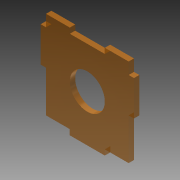
# Autodesk Inventor part: SideB
Saved by Autodesk Inventor 2014 (Build 180170000, 170)
## iProperties
Created: 2014-11-21
Part Number: SideB
Material: Generic
Document SubType Name: Modeling
Designer: JLM
Density: 1 g/cm^3
Appearance: Default
Author: JLM
Autodesk Inventor part; units mm, degrees
ref_plane "YZ Plane" through (0, 0, 0) normal (1, 0, 0) x (0, 1, 0)
ref_plane "XZ Plane" through (0, 0, 0) normal (0, 1, 0) x (-1, 0, 0)
ref_plane "XY Plane" through (0, 0, 0) normal (0, 0, 1) x (1, 0, 0)
sketch "Sketch1" plane through (0, 0, 0) normal (0, 0, 1) x (1, 0, 0)
  line L0 (-25.4, -25.4) -> (25.4, -25.4)
  line L1 (25.4, -25.4) -> (25.4, 25.4)
  line L2 (25.4, 25.4) -> (-25.4, 25.4)
  line L3 (-25.4, 25.4) -> (-25.4, -25.4)
  line L4 (-25.4, -25.4) -> (25.4, 25.4) construction
  line L5 (25.4, -25.4) -> (-25.4, 25.4) construction
  point P0 (0, 0)
  dimension "d0" = 50.8
  dimension "d1" = 50.8
  constraints: 12 end point, 2 midpoint, 2 parallel, 1 horizontal, 1 perpendicular
  measures "d0" distance of L2.end L1.end
  measures "d1" distance of L1.end L0.end
extrude "Extrusion1" add sketch "Sketch1" against normal blind 2.921
sketch "Sketch4" plane through (0, 0, 0) normal (0, 0, 1) x (1, 0, 0)
  line L0 (-25.4, -25.4) -> (-9.525, -25.4)
  line L1 (-9.525, -25.4) -> (-9.525, -22.479)
  line L2 (-9.525, -22.479) -> (-25.4, -22.479)
  line L3 (-25.4, -22.479) -> (-25.4, -25.4)
  line L4 (25.4, 25.4) -> (-25.4, 25.4) projected
  line L5 (-25.4, 25.4) -> (-25.4, -25.4) projected
  line L6 (-9.525, 25.4) -> (9.525, 25.4)
  line L7 (9.525, 25.4) -> (9.525, 22.479)
  line L8 (9.525, 22.479) -> (-9.525, 22.479)
  line L9 (-9.525, 22.479) -> (-9.525, 25.4)
  line L10 (-25.4, -25.4) -> (-22.479, -25.4)
  line L11 (-22.479, -25.4) -> (-22.479, 0)
  line L12 (-22.479, 0) -> (-25.4, 0)
  line L13 (-25.4, 0) -> (-25.4, -25.4)
  line L14 (-25.4, 25.4) -> (-22.479, 25.4)
  line L15 (-22.479, 25.4) -> (-22.479, 19.05)
  line L16 (-22.479, 19.05) -> (-25.4, 19.05)
  line L17 (-25.4, 19.05) -> (-25.4, 25.4)
  line L18 (0, -3.175) -> (0, -6.3407)
  line L19 (25.4, -25.4) -> (9.525, -25.4)
  line L20 (9.525, -25.4) -> (9.525, -22.479)
  line L21 (9.525, -22.479) -> (25.4, -22.479)
  line L22 (25.4, -22.479) -> (25.4, -25.4)
  line L23 (25.4, 25.4) -> (25.4, -25.4)
  line L24 (9.525, 22.479) -> (9.525, 25.4)
  line L25 (25.4, -25.4) -> (22.479, -25.4)
  line L26 (22.479, -25.4) -> (22.479, 0)
  line L27 (22.479, 0) -> (25.4, 0)
  line L28 (25.4, 0) -> (25.4, -25.4)
  line L29 (25.4, 25.4) -> (22.479, 25.4)
  line L30 (22.479, 25.4) -> (22.479, 19.05)
  line L31 (22.479, 19.05) -> (25.4, 19.05)
  line L32 (25.4, 19.05) -> (25.4, 25.4)
  point P0 (0, 0)
  point P1 (25.4, 0.1976)
  dimension "d16" = 2.921
  dimension "d37" = 9.525
  dimension "d38" = 15.875
  dimension "d44" = 2.921
  dimension "d45" = 19.05
  dimension "d46" = 15.875
  dimension "d53" = 25.4
  dimension "d54" = 19.05
  dimension "d55" = 2.921
  dimension "d56" = 2.921
  constraints: 62 end point, 11 symmetric about line, 9 parallel, 4 horizontal, 4 perpendicular, 2 point on line
  measures "d16" distance of L0.end L1.end
  measures "d37" distance from line of point (0, 0) L1
  measures "d38" distance of L0.start L0.end
  measures "d44" distance of L8.end L6.start
  measures "d45" distance of L7.end L8.end
  measures "d46" distance between parallel lines of L5 L9
  measures "d53" distance of L11.end L10.end
  measures "d54" distance between parallel lines of L12 L16
  measures "d55" distance of L15.end L16.end
  measures "d56" distance of L11.end L12.end
extrude "Extrusion5" cut sketch "Sketch4" against normal blind 25.4
hole "Hole1" at (0, 0, 0) direction (0, 0, -1) diameter 19.05 end through all
equation "\"d38\" = -d37 + 0.5 * d0"
equation "\"d44\" = d16"
equation "\"d45\" = d42"
equation "\"d46\" = d38"
equation "\"d55\" = d16"
equation "\"d56\" = d16"
equation "\"d48\" = 0.5 * d0"
equation "\"d42\" = 2 * d37"
body "Solid1"
